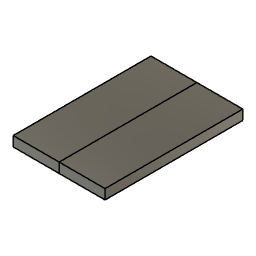
_Snap Joint (Autodesk Fusion 360 design; units mm, degrees)
part number: 2025-05-23-21-47-17-750
Autodesk Fusion 360 part; units mm, degrees
note: some values were not read from the file. Set by a fixed rule: which face or edge a step refers to.
sketch "Sketch1" plane through (0, 0, 0) normal (0, 0, 1) x (1, 0, 0)
  line L0 (0, 0) -> (84, 0)
  line L1 (84, 0) -> (84, 28)
  line L2 (84, 28) -> (0, 28)
  line L3 (0, 28) -> (0, 0)
  dimension "d1" = 84
  dimension "d2" = 28
  constraint horizontal L0
  constraint vertical L1
  constraint horizontal L2
  constraint vertical L3
  constraint coincident L0.start L3.end
  measures "d1" distance of L0.start L0.end
  measures "d2" distance of L0.start L2.end
extrude "Extrude1" add sketch "Sketch1" against normal blind 4.5 makes body 1
ref_plane "WorkPlane1" through (42, 14, -2.25) normal (0, 0, 1) x (1, 0, 0)
sketch "Sketch2" plane through (0, 0, -2.25) normal (0, 0, 1) x (1, 0, 0)
  line L0 (0, 19) -> (-5, 19)
  line L1 (-5, 19) -> (-5, 19.4)
  line L2 (-5.6, 20) -> (-7.4, 20)
  line L3 (-8, 19.4) -> (-8, 18.8178)
  line L4 (0, 17.5) -> (1.4347, 17.5)
  line L5 (2.3966, 17.9028) -> (2.4415, 17.9484)
  line L6 (2.8295, 18.8956) -> (2.8295, 19)
  line L7 (2.8295, 19) -> (2.8295, 19.8)
  line L8 (2.8295, 19.8) -> (0, 19.8)
  line L9 (0, 19.8) -> (0, 19)
  arc A0 (2.4415, 17.9484) -> (2.8295, 18.8956) centre (1.4795, 18.8956) ccw
  arc A1 (1.4347, 17.5) -> (2.3966, 17.9028) centre (1.4347, 18.85) ccw
  line L10 (-5, 18) -> (0, 17.5)
  line L11 (-8, 18.8178) -> (-8.4, 18.8178)
  line L12 (-10, 17.2178) -> (-10, 16.925)
  line L13 (-7.6, 18) -> (-5, 18)
  arc A2 (-8.4, 18.8178) -> (-10, 17.2178) centre (-8.4, 17.2178) ccw
  arc A3 (-7.6, 18) -> (-9.2, 16.4) centre (-7.6, 16.4) ccw
  arc A4 (-10, 16.925) -> (-9.66, 16.245) centre (-9.15, 16.925) ccw
  line L14 (-9.3021, 16.1156) -> (-9.3552, 16.0977)
  line L15 (-9.66, 16.245) -> (-9.4931, 16.1198)
  line L16 (-9.2, 16.2577) -> (-9.2, 16.4)
  arc A5 (-9.4931, 16.1198) -> (-9.3552, 16.0977) centre (-9.4031, 16.2398) ccw
  arc A6 (-9.3021, 16.1156) -> (-9.2, 16.2577) centre (-9.35, 16.2577) ccw
  arc A7 (-7.4, 20) -> (-8, 19.4) centre (-7.4, 19.4) ccw
  arc A8 (-5, 19.4) -> (-5.6, 20) centre (-5.6, 19.4) ccw
  dimension "d5" = 1.35
  dimension "d7" = 1.6
  dimension "d8" = 0.85
  dimension "d9" = 0.15
  dimension "d10" = 0.6
  constraint horizontal L0
  constraint perpendicular L0 L1
  constraint perpendicular L1 L2
  constraint perpendicular L2 L3
  constraint horizontal L4
  constraint perpendicular L4 L6
  constraint perpendicular L4 L7
  constraint perpendicular L6 L8
  constraint perpendicular L0 L9
  constraint tangent L5 A0
  constraint tangent L6 A0
  constraint tangent L4 A1
  constraint tangent L5 A1
  constraint equal A0 A1
  constraint perpendicular L3 L11
  constraint perpendicular L11 L12
  constraint tangent L11 A2
  constraint tangent L12 A2
  constraint tangent L13 A3
  constraint equal A2 A3
  constraint tangent L12 A4
  constraint tangent A4 L15
  constraint tangent A3 L16
  constraint tangent L14 A5
  constraint tangent L15 A5
  constraint tangent L14 A6
  constraint tangent L16 A6
  constraint equal A5 A6
  constraint tangent L2 A7
  constraint tangent L3 A7
  constraint tangent L1 A8
  constraint tangent L2 A8
  constraint equal A7 A8
  measures "d5" radius of A0
  measures "d7" radius of A2
  measures "d8" radius of A4
  measures "d9" radius of A5
  measures "d10" radius of A7
ref_plane "WorkPlane2" through (42, 14, -2.25) normal (0, 0, 1) x (1, 0, 0)
extrude "Extrude2" add sketch "Sketch2" along normal mid plane 4 separate body makes body 2
extrude "Extrude3" add 1 faces at (28, 9.3333, -4.5) along direction (0, 0, -1) blind 1.5 on bodies 1 bodies 1
move_body "Move1" bodies 2 to x (1, 0, 0) y (0, 1, 0) z (0, 0, 1) at (0, 0, -0.75)
extrude "Extrude4" add 1 faces at (28, 0, -2) along direction (0, -1, 0) blind 28 on bodies 1 bodies 1
extrude "Extrude5" add 1 faces at (56, 28, -2) along direction (0, 1, 0) blind 28 on bodies 1 bodies 1
extrude "Extrude6" cut 1 faces at (84, 0, -2) along direction (-1, 0, 0) blind 56 on bodies 1 bodies 1
ref_plane "WorkPlane4" through (14, 14, -3) normal (0, -1, 0) x (0, 0, -1)
move_body "Move2" bodies 2 to x (1, 0, 0) y (0, 1, 0) z (0, 0, 1) at (0, 20, 0)
mirror "Mirror1" about plane through (14, 14, -3) normal (0, -1, 0) of bodies 2 makes body 3
ref_plane "WorkPlane5" through (14, 14, -3) normal (0, 0, 1) x (1, 0, 0)
sketch "Sketch5" plane through (0, 0, -3) normal (0, 0, 1) x (1, 0, 0)
  line L0 (0, 39.8) -> (3.4, 39.8)
  line L1 (3.4, 39.8) -> (3.4, 36.9)
  line L2 (3.4, 36.9) -> (0, 36.9)
  line L3 (0, 36.9) -> (0, 39.8)
  dimension "d23" = 2.9
  constraint horizontal L0
  constraint vertical L1
  constraint horizontal L2
  constraint vertical L3
  measures "d23" distance of L0.start L2.end
extrude "Extrude7" cut sketch "Sketch5" along normal mid plane 4 bodies 1
mirror "Mirror2" about plane through (14, 14, -3) normal (0, -1, 0) of "Extrude7"
combine "Combine1" operation add target body 1 tool bodies 2 3 keep tools
sketch "Sketch6" plane through (0, 0, 0) normal (-1, 0, 0) x (0, -1, 0)
  line L0 (11, -5) -> (9.5, -5)
  line L1 (9.5, -5) -> (8.9, -5)
  line L2 (8.9, -5) -> (8.9, -1)
  line L3 (8.9, -1) -> (9.5, -1)
  line L4 (9.5, -1) -> (11, -1)
  line L5 (11, -1) -> (11, -5)
  line L6 (-36.9, -5) -> (-37.5, -5)
  line L7 (-37.5, -5) -> (-39, -5)
  line L8 (-39, -5) -> (-39, -1)
  line L9 (-39, -1) -> (-37.5, -1)
  line L10 (-37.5, -1) -> (-36.9, -1)
  line L11 (-36.9, -1) -> (-36.9, -5)
  line L12 (28, 0) -> (-56, 0)
  line L13 (-56, 0) -> (-56, -6)
  line L14 (-56, -6) -> (28, -6)
  line L15 (28, -6) -> (28, 0)
  line L16 (25, -4) -> (19, -4)
  line L17 (19, -4) -> (19, -2)
  line L18 (19, -2) -> (25, -2)
  line L19 (25, -2) -> (25, -4)
  constraint horizontal L16
  constraint vertical L17
  constraint horizontal L18
  constraint vertical L19
extrude "Extrude8" add sketch "Sketch6" along normal blind 5 contours L16 L17 L18 L19 bodies 1
mirror "Mirror3" about plane through (14, 14, -3) normal (0, -1, 0) of "Extrude8"
sketch "Sketch7" plane through (0, 0, 0) normal (0, 0, 1) x (1, 0, 0)
  line L0 (0, 56) -> (-28, 56)
  line L1 (-28, 56) -> (-28, -28)
  line L2 (-28, -28) -> (0, -28)
  line L3 (0, -28) -> (0, 56)
  dimension "d32" = 28
  dimension "d33" = 84
  constraint horizontal L0
  constraint vertical L1
  constraint horizontal L2
  constraint vertical L3
  measures "d32" distance of L0.start L0.end
  measures "d33" distance of L0.start L2.end
extrude "Extrude9" add sketch "Sketch7" against normal blind 6 separate body makes body 4
combine "Combine2" operation cut target body 4 tool bodies 1 keep tools
ref_plane "WorkPlane7" through (-14, 14, -3) normal (0, 0, 1) x (1, 0, 0)
sketch "Sketch8" plane through (0, 0, -3) normal (0, 0, 1) x (1, 0, 0)
  line L0 (-10.6, 39.2) -> (-10.6, 34.7576)
  line L1 (-10.6, 34.7576) -> (0, 34.7576)
  line L2 (0, 34.7576) -> (0, 39.2)
  line L3 (-4.9, 39.2) -> (-4.9, 39.4)
  line L4 (-5.6, 40.1) -> (-7.4, 40.1)
  line L5 (-8.1, 39.4) -> (-8.1, 39.2)
  arc A0 (-4.9, 39.4) -> (-5.6, 40.1) centre (-5.6, 39.4) ccw
  arc A1 (-7.4, 40.1) -> (-8.1, 39.4) centre (-7.4, 39.4) ccw
  line L6 (0, 39.2) -> (-4.9, 39.2)
  line L7 (-8.1, 39.2) -> (-10.6, 39.2)
  dimension "d36" = 10.6
  dimension "d37" = 0.7
  constraint vertical L0
  constraint horizontal L1
  constraint vertical L2
  constraint perpendicular L3 L4
  constraint perpendicular L4 L5
  constraint tangent L3 A0
  constraint tangent L4 A0
  constraint tangent L4 A1
  constraint tangent L5 A1
  constraint equal A0 A1
  constraint perpendicular L3 L6
  constraint perpendicular L0 L7
  measures "d36" distance of L2.end L0.start
  measures "d37" radius of A0
extrude "Extrude10" cut sketch "Sketch8" along normal mid plane 4.2 bodies 4
ref_plane "WorkPlane8" through (-14, 14, -3) normal (0, 1, 0) x (1, 0, 0)
mirror "Mirror4" about plane through (14, 14, -3) normal (0, -1, 0) of "Extrude10"
extrude "Extrude11" cut 1 faces at (-5.1667, 36.2384, -0.9) along direction (0, 0, 1) blind 0.1 on bodies 4 bodies 4
extrude "Extrude12" cut 1 faces at (-5.1667, 36.2384, -5.1) along direction (0, 0, -1) blind 0.1 on bodies 4 bodies 4
mirror "Mirror5" about plane through (14, 14, -3) normal (0, -1, 0) of "Extrude11", "Extrude12"
move_face "OffsetFaces2" offset -0.2 5 faces at (-5, 51, -3.3333) (-1.6667, 47, -3.3333) (-1.6667, 49, -2) (-1.6667, 53, -2.6667) (-1.6667, 51, -4) on bodies 4
move_face "OffsetFaces3" offset -0.2 5 faces at (-1.6667, -23, -4) (-3.3333, -19, -2.6667) (-5, -21, -2.6667) (-1.6667, -25, -2.6667) (-1.6667, -21, -2) on bodies 4
hidden bodies 2 3
named bodies: "Male Joint", "Female Joint"
